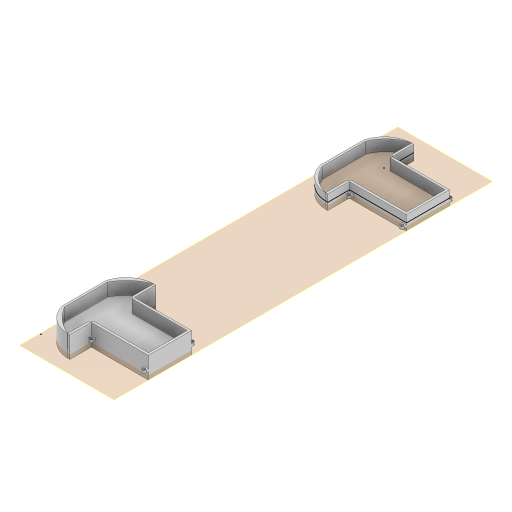
# Autodesk Inventor part: Part1
Saved by Autodesk Inventor 2024.3 (Build 283343000, 343)
## iProperties
Created: 2025-09-23
Part Number: Part1
Material: Generic
Document SubType Name: Modeling
Designer: danie
Density: 1 g/cm^3
Appearance: Default
Author: danie
Autodesk Inventor part; units mm, degrees
ref_plane "YZ Plane" through (0, 0, 0) normal (1, 0, 0) x (0, 1, 0)
ref_plane "XZ Plane" through (0, 0, 0) normal (0, 1, 0) x (-1, 0, 0)
ref_plane "XY Plane" through (0, 0, 0) normal (0, 0, 1) x (1, 0, 0)
sketch "Sketch1" plane through (0, 0, 0) normal (0, 1, 0) x (-1, 0, 0)
  line L0 (-60.8639, 0) -> (-200, 0)
  line L1 (-200, 0) -> (-200, -200)
  line L2 (-200, -200) -> (0, -200)
  line L3 (0, -200) -> (0, 0)
  line L4 (0, -200) -> (-200, -200)
  line L5 (-200, -200) -> (-200, -400)
  line L6 (-200, -400) -> (0, -400)
  line L7 (0, -400) -> (0, -200)
  line L8 (-60.8639, 0) -> (-67, 0)
  line L9 (0, -200) -> (0, -100)
  line L10 (0, -50) -> (0, -100)
  line L11 (0, -100) -> (0, -50)
  line L12 (0, -50) -> (0, -150)
  line L13 (0, -150) -> (-67, -150)
  line L14 (0, -50) -> (-67, -50)
  line L15 (-14.5617, -10.867) -> (0, 0)
  line L16 (-67, -150) -> (0, -200)
  arc A0 (0, -50) -> (-67, 0) centre (-63.932, -65.7788) ccw
  line L17 (0, -200) -> (15.754, -200)
  line L18 (15.754, -200) -> (0, -200)
  line L19 (0, -200) -> (0, -184.246)
  line L20 (0, -184.246) -> (-21.1104, -184.246)
  line L21 (-21.1104, -184.246) -> (-21.1104, -200)
  arc A1 (-67, -200) -> (0, -150) centre (-63.9339, -134.2186) ccw
  line L22 (-67, -50) -> (-200, -50)
  line L23 (-67, -150) -> (-200, -150)
  line L24 (-67, 0) -> (-67, -50)
  line L25 (-67, -150) -> (-67, -200)
  line L26 (-200, -800) -> (-200, -600)
  line L27 (0, -750) -> (0, -700)
  line L28 (0, -750) -> (0, -650)
  line L29 (0, -650) -> (-67, -650)
  line L30 (0, -750) -> (-67, -750)
  line L31 (-67, -650) -> (0, -600)
  arc A2 (-67, -800) -> (0, -750) centre (-63.932, -734.2212) ccw
  arc A3 (0, -650) -> (-67, -600) centre (-63.9339, -665.7814) ccw
  line L32 (-67, -750) -> (-200, -750)
  line L33 (-67, -650) -> (-200, -650)
  line L34 (-67, -800) -> (-67, -750)
  line L35 (-67, -650) -> (-67, -600)
  point P0 (-60.8677, -200)
  dimension "d0" = 200
  dimension "d1" = 200
  dimension "d2" = 200
  dimension "d3" = 200
  dimension "d4" = 67
  dimension "d5" = 100
  dimension "d6" = 50
  dimension "d7" = 100
  dimension "d8" = 15.754
  dimension "d9" = 15.754
  constraints: 72 end point, 14 symmetric about line, 13 perpendicular, 10 point on circle, 9 point on line, 4 centre point, 4 parallel, 2 collinear, 2 horizontal, 2 midpoint, 2 other
  measures "d0" distance of L2.end L1.end
  measures "d1" distance of L1.end L0.end
  measures "d2" distance of L6.end L5.end
  measures "d3" distance of L5.end L4.end
  measures "d4" distance of L3.end L8.end
  measures "d5" distance of L3.end L9.end
  measures "d6" distance of L10.start L9.end
  measures "d7" distance of L10.start L12.end
  measures "d8" distance of L2.end L17.end
  measures "d9" distance of L2.end L19.end
extrude "Extrusion1" add sketch "Sketch1" along normal blind 50 contours A0 L14 L24 L0 | L3 L13 L23 L1 L22 L14 | A1 L16 L13 | L16 A1 L2 L25 | L26 L33 L29 L28 L27 L30 L32 | L30 A2 L34 | L31 A3 L29 | L35 A3 L31
sketch "Sketch2" plane through (0, 50, 0) normal (0, 1, 0) x (1, 0, 0)
  line L0 (67, 50) -> (200, 50) projected
  line L1 (200, 50) -> (200, 150)
  line L2 (200, 150) -> (67, 150)
  line L3 (67, 150) -> (67, 199.2984)
  line L4 (67, 199.2984) -> (67, 200.0458)
  line L5 (0, 150) -> (0, 50) projected
  line L6 (0, 50) -> (0, 150)
  line L7 (67, 50) -> (200, 50)
  arc A0 (0, 50) -> (63.932, 0) centre (63.792, 65.694) ccw
  arc A1 (60.8677, 200) -> (0, 150) centre (63.9339, 134.2186) ccw projected
  arc A2 (67, 200.0458) -> (0, 150) centre (64.0367, 134.1412) ccw
  line L8 (107.1865, 50) -> (107.1865, 55)
  line L9 (107.1865, 55) -> (67, 55)
  line L10 (200, 55) -> (195, 55)
  line L11 (195, 150) -> (195, 145)
  line L12 (195, 145) -> (67, 145)
  line L13 (67, 145) -> (67, 55)
  line L14 (67, 55) -> (195, 55)
  line L15 (195, 55) -> (195, 145)
  line L16 (0, 102.5601) -> (5, 102.5601)
  line L17 (5, 102.5601) -> (5, 150)
  line L18 (67, 150) -> (67, 200) projected
  line L19 (67, 150) -> (62, 150)
  line L20 (62, 150) -> (5, 150)
  line L21 (62, 150) -> (62, 145)
  line L22 (62, 145) -> (72.629, 145)
  line L23 (67, 50) -> (62, 50)
  line L24 (62, 50) -> (62, 55)
  line L25 (62, 50) -> (5, 50)
  line L26 (5, 50) -> (5, 104.6986)
  line L27 (67, 55) -> (62, 55)
  line L28 (62, 50) -> (67, 55)
  line L29 (67, 145) -> (62, 150)
  line L30 (67, 200) -> (62.0007, 200.081)
  line L31 (62.0007, 200.081) -> (62, 150)
  arc A3 (62.0007, 200.081) -> (5, 150) centre (102.4081, 96.6117) ccw
  line L32 (62.0007, 50.0007) -> (62.0007, 0.0243)
  arc A4 (5, 50) -> (62.0007, 0.0243) centre (106.1149, 107.8339) ccw
  point P0 (0, 0)
  point P1 (62.0007, 50)
  dimension "d12" = 5
  dimension "d13" = 5
  dimension "d14" = 5
  dimension "d15" = 5
  dimension "d16" = 5
  dimension "d17" = 5
  dimension "d18" = 5
  constraints: 60 end point, 12 perpendicular, 10 point on circle, 9 point on line, 4 centre point, 4 horizontal, 2 collinear, 2 parallel, 2 vertical
  measures "d12" distance of L8.start L8.end
  measures "d13" distance of L10.start L10.end
  measures "d14" distance of L11.start L11.end
  measures "d15" distance of L16.start L16.end
  measures "d16" distance of L2.end L19.end
  measures "d17" distance of L0.start L23.end
  measures "d18" distance of L18.end L30.end
extrude "Extrusion2" cut sketch "Sketch2" against normal blind 30 contours L25 L26 L17 L20 L21 L22 L13 L27 L24 | L32 A4 L25 | L24 L27 L28 | L9 L13 L12 L15 L14 | L22 L21 L29 | L20 A3 L31
ref_plane "Work Plane1" through (0, 10, 0) normal (0, 1, 0) x (1, 0, 0)
sketch "Sketch3" plane through (0, 20, 0) normal (0, 1, 0) x (1, 0, 0)
  line L0 (67, 150) -> (200, 150) projected
  line L1 (200, 150) -> (200, 50) projected
  line L2 (200, 50) -> (67, 50) projected
  line L3 (67, 50) -> (67, 0) projected
  line L4 (67, 0) -> (60.8639, 0) projected
  arc A0 (0, 50) -> (60.8639, 0) centre (63.932, 65.7788) ccw projected
  line L5 (0, 50) -> (0, 150) projected
  arc A1 (60.8677, 200) -> (0, 150) centre (63.9339, 134.2186) ccw projected
  line L6 (60.8677, 200) -> (61.7939, 200) projected
  arc A2 (61.7939, 200) -> (5, 150) centre (102.4081, 96.6117) ccw projected
  line L7 (5, 150) -> (5, 50) projected
  arc A3 (5, 50) -> (62.0007, 0.0243) centre (106.1149, 107.8339) ccw projected
  line L8 (62.0007, 0.0243) -> (62.0007, 50) projected
  line L9 (62.0007, 50) -> (62, 50) projected
  line L10 (62, 50) -> (67, 55) projected
  line L11 (67, 55) -> (195, 55) projected
  line L12 (195, 55) -> (195, 145) projected
  line L13 (195, 145) -> (67, 145) projected
  line L14 (67, 145) -> (62, 150) projected
  line L15 (62, 150) -> (62.0007, 200) projected
  line L16 (61.7939, 200) -> (62.0007, 200) projected
  line L17 (67, 200) -> (67, 150) projected
  line L18 (62.0007, 200) -> (67, 200) projected
  arc A4 (0, 650) -> (67, 600) centre (63.9339, 665.7814) ccw projected
  line L19 (0, 650) -> (0, 750) projected
  arc A5 (67, 800) -> (0, 750) centre (63.932, 734.2212) ccw projected
  line L20 (67, 800) -> (67, 750) projected
  line L21 (67, 750) -> (200, 750) projected
  line L22 (200, 750) -> (200, 650) projected
  line L23 (200, 650) -> (67, 650) projected
  line L24 (67, 650) -> (67, 600) projected
  line L25 (67, 150) -> (200, 150) projected
  line L26 (200, 150) -> (200, 50) projected
  line L27 (200, 50) -> (67, 50) projected
  line L28 (67, 50) -> (67, 0) projected
  line L29 (67, 0) -> (60.8639, 0) projected
  arc A6 (0, 50) -> (60.8639, 0) centre (63.932, 65.7788) ccw projected
  line L30 (0, 50) -> (0, 150) projected
  arc A7 (60.8677, 200) -> (0, 150) centre (63.9339, 134.2186) ccw projected
  line L31 (60.8677, 200) -> (61.7939, 200) projected
  arc A8 (61.7939, 200) -> (5, 150) centre (102.4081, 96.6117) ccw projected
  line L32 (5, 150) -> (5, 50) projected
  arc A9 (5, 50) -> (62.0007, 0.0243) centre (106.1149, 107.8339) ccw projected
  line L33 (62.0007, 0.0243) -> (62.0007, 50) projected
  line L34 (62.0007, 50) -> (62, 50) projected
  line L35 (62, 50) -> (67, 55) projected
  line L36 (67, 55) -> (195, 55) projected
  line L37 (195, 55) -> (195, 145) projected
  line L38 (195, 145) -> (67, 145) projected
  line L39 (67, 145) -> (62, 150) projected
  line L40 (62, 150) -> (62.0007, 200) projected
  line L41 (61.7939, 200) -> (62.0007, 200) projected
  line L42 (67, 200) -> (67, 150) projected
  line L43 (62.0007, 200) -> (67, 200) projected
  arc A10 (0, 650) -> (67, 600) centre (63.9339, 665.7814) ccw projected
  line L44 (0, 650) -> (0, 750) projected
  arc A11 (67, 800) -> (0, 750) centre (63.932, 734.2212) ccw projected
  line L45 (67, 800) -> (67, 750) projected
  line L46 (67, 750) -> (200, 750) projected
  line L47 (200, 750) -> (200, 650) projected
  line L48 (200, 650) -> (67, 650) projected
  line L49 (67, 650) -> (67, 600) projected
  line L50 (67, 50) -> (200, 50) projected
  line L51 (67, 50) -> (77, 50)
  line L52 (77, 50) -> (77, 40)
  line L53 (77, 40) -> (67, 40)
  line L54 (67, 40) -> (67, 50)
  line L55 (200, 50) -> (190, 50)
  line L56 (190, 50) -> (190, 40)
  line L57 (190, 40) -> (200, 40)
  line L58 (200, 40) -> (200, 50)
  line L59 (200, 50) -> (200, 150) projected
  line L60 (200, 150) -> (190, 150)
  line L61 (190, 150) -> (190, 160)
  line L62 (190, 160) -> (200, 160)
  line L63 (200, 160) -> (200, 150)
  line L64 (67, 150) -> (77, 150)
  line L65 (77, 150) -> (77, 160)
  line L66 (77, 160) -> (67, 160)
  line L67 (67, 160) -> (67, 150)
  circle A12 centre (72, 45) radius 5
  circle A13 centre (195, 45) radius 5
  circle A14 centre (195, 155) radius 5
  circle A15 centre (72, 155) radius 5
  point P0 (0, 0)
  point P1 (67, 45)
  point P2 (77, 45)
  point P3 (190, 45)
  point P4 (200, 45)
  point P5 (190, 155)
  point P6 (200, 155)
  point P7 (77, 155)
  point P8 (67, 155)
  dimension "d21" = 10
  dimension "d22" = 10
  dimension "d23" = 10
  dimension "d24" = 10
  dimension "d25" = 10
  dimension "d26" = 10
  dimension "d27" = 10
  constraints: 32 end point, 8 parallel, 4 centre point, 4 horizontal, 4 perpendicular
  measures "d21" distance of L52.end L53.end
  measures "d22" distance of L51.end L52.end
  measures "d23" distance of L57.end L56.end
  measures "d24" distance of L56.end L55.end
  measures "d25" distance of L61.end L62.end
  measures "d26" distance of L60.end L61.end
  measures "d27" distance of L66.end L65.end
extrude "Extrusion3" add sketch "Sketch3" along normal mid plane 5.75 contours L0 A15 L65 | L61 A14 L0 | L0 L17 A15 | A15 | A14 L63 L0 | A14 | L58 A13 L2 | A13 L56 L2 | A13 | L52 A12 L2 | A12 L3 L2 | A12
sketch "Sketch4" plane through (0, 22.875, 0) normal (0, 1, 0) x (1, 0, 0)
  circle A0 centre (72, 44.2688) radius 3.375
  arc A1 (190, 45) -> (200, 45) centre (195, 45) ccw projected
  line L0 (195, 40) -> (195, 44.2688)
  circle A2 centre (195, 44.2688) radius 3.375
  arc A3 (200, 155) -> (190, 155) centre (195, 155) ccw projected
  line L1 (195, 160) -> (195, 155.731)
  circle A4 centre (195, 155.731) radius 2.875
  circle A5 centre (195, 155.731) radius 3.375
  arc A6 (77, 155) -> (67, 155) centre (72, 155) ccw projected
  line L2 (72, 160) -> (72, 155.731)
  circle A7 centre (72, 155.731) radius 3.375
  point P0 (0, 0)
  dimension "d30" = 6.75
  dimension "d31" = 4.269
  dimension "d32" = 5.75
  dimension "d33" = 6.75
  constraints: 6 end point, 5 centre point, 4 coincident, 3 point on circle, 3 vertical
  measures "d30" diameter of A0
  measures "d31" distance of L1.start L1.end
  measures "d32" diameter of A4
  measures "d33" diameter of A5
extrude "Extrusion4" cut sketch "Sketch4" against normal blind 5.75 contours A0 | A2 | A4 | A5 | A7
thread "Thread1" size "M7x1" class "6H" standard "ANSI Metric M Profile" full length
thread "Thread2" size "M7x1" class "6H" standard "ANSI Metric M Profile" full length
thread "Thread3" size "M7x1" class "6H" standard "ANSI Metric M Profile" full length
thread "Thread4" size "M7x1" class "6H" standard "ANSI Metric M Profile" full length
sketch "Sketch5" plane through (0, 17.125, 0) normal (0, -1, 0) x (1, 0, 0)
  line L0 (200, -750) -> (67, -750)
  line L1 (67, -750) -> (200, -750)
  line L2 (200, -750) -> (200, -650.0001)
  line L3 (200, -650.0001) -> (67, -650.0001)
  line L4 (67, -600) -> (67, -650)
  line L5 (0, -750) -> (0, -650)
  arc A0 (67, -600) -> (0, -650) centre (63.2865, -664.914) ccw
  arc A1 (0, -750) -> (67, -800) centre (63.932, -734.2212) ccw
  arc A2 (0, -750) -> (67, -800) centre (63.932, -734.2212) ccw
  line L6 (0, -650) -> (0, -750)
  line L7 (67, -750) -> (67, -800)
  line L8 (67, -600) -> (67, -650)
  point P0 (0, 0)
  constraints: 18 end point, 6 point on circle, 3 centre point
sketch "Sketch6" plane through (0, 50, 0) normal (0, 1, 0) x (1, 0, 0)
  arc A0 (0, 650) -> (67, 600) centre (63.9339, 665.7814) ccw projected
  line L0 (0, 750) -> (0, 650) projected
  line L1 (0, 650) -> (0, 750)
  line L2 (67, 650) -> (200, 650) projected
  line L3 (67, 650) -> (200, 650)
  line L4 (200, 650) -> (200, 750)
  line L5 (200, 750) -> (67, 750)
  line L6 (67, 750) -> (67, 800)
  line L7 (67, 600) -> (67, 650) projected
  line L8 (67, 650) -> (67, 600)
  arc A1 (0, 650) -> (67, 600) centre (63.9339, 665.7814) ccw
  arc A2 (67, 800) -> (0, 750) centre (63.932, 734.2212) ccw projected
  arc A3 (67, 800) -> (0, 750) centre (63.932, 734.2212) ccw
  point P0 (0, 0)
  dimension "d44" = 50
  constraints: 12 end point, 4 point on circle, 3 perpendicular, 2 centre point, 1 collinear, 1 concentric, 1 horizontal, 1 vertical
  measures "d44" distance of L5.end L6.end
extrude "Extrusion5" cut sketch "Sketch6" against normal blind 16.5
sketch "Sketch7" plane through (0, 33.5, 0) normal (0, 1, 0) x (1, 0, 0)
  line L0 (200, 750) -> (67, 750) projected
  line L1 (200, 750) -> (200, 745)
  line L2 (0, 750) -> (0, 650) projected
  line L3 (200, 745) -> (195, 745)
  line L4 (67, 650) -> (200, 650) projected
  line L5 (195, 650) -> (195, 655)
  line L6 (195, 655) -> (67, 655)
  line L7 (195, 655) -> (195, 745)
  line L8 (200, 650) -> (200, 750) projected
  line L9 (195, 745) -> (67, 745)
  line L10 (67, 745) -> (67, 655)
  line L11 (67, 800.7968) -> (62, 800.7968)
  line L12 (62, 800.7968) -> (62, 600)
  line L13 (67, 650) -> (67, 655)
  line L14 (67, 655) -> (62, 650)
  line L15 (67, 750) -> (62, 755)
  line L16 (0, 750) -> (5, 750)
  arc A0 (67, 800) -> (0, 750) centre (63.932, 734.2212) ccw projected
  line L17 (62, 800.0432) -> (65.8623, 800.1565)
  line L18 (65.8623, 800.1565) -> (67, 800)
  line L19 (67, 800) -> (62, 800.0432)
  line L20 (67, 800) -> (67, 750)
  line L21 (0, 750) -> (0, 650)
  line L22 (0, 650) -> (5, 650)
  line L23 (5, 650) -> (5, 750)
  arc A1 (62, 800.0432) -> (5, 750) centre (81.2834, 720.5955) ccw
  line L24 (62, 650) -> (62, 600)
  arc A2 (0, 650) -> (67, 600) centre (63.9339, 665.7814) ccw projected
  line L25 (62, 600) -> (67, 600)
  line L26 (67, 600) -> (67, 600)
  line L27 (67, 650) -> (67, 600)
  arc A3 (5, 650) -> (62, 600) centre (82.4475, 680.8001) ccw
  line L28 (67, 750) -> (67, 650)
  point P0 (0, 0)
  dimension "d47" = 5
  dimension "d48" = 5
  dimension "d49" = 5
  dimension "d50" = 5
  dimension "d51" = 5
  constraints: 50 end point, 8 perpendicular, 5 point on circle, 5 point on line, 4 horizontal, 4 parallel, 2 centre point, 2 vertical, 1 tangent
  measures "d47" distance of L0.start L1.end
  measures "d48" distance of L1.end L3.end
  measures "d49" distance of L5.start L5.end
  measures "d50" distance of L11.start L11.end
  measures "d51" distance of L2.start L16.end
extrude "Extrusion6" cut sketch "Sketch7" against normal blind 25.75 contours L28 L10 L14 L12 L15 | L12 A3 L23 A1 | L9 L7 L6 L10
sketch "Sketch8" plane through (0, 10, 0) normal (0, 1, 0) x (1, 0, 0)
  line L0 (61.7939, 200) -> (62.0007, 200) projected
  arc A0 (61.7939, 200) -> (5, 150) centre (102.4081, 96.6117) ccw projected
  line L1 (5, 50) -> (5, 150) projected
  arc A1 (5, 50) -> (62.0007, 0.0243) centre (106.1149, 107.8339) ccw projected
  line L2 (62.0007, 50) -> (62.0007, 0.0243) projected
  line L3 (62, 50) -> (62.0007, 50) projected
  line L4 (67, 55) -> (62, 50) projected
  line L5 (195, 55) -> (67, 55) projected
  line L6 (195, 145) -> (195, 55) projected
  line L7 (67, 145) -> (195, 145) projected
  line L8 (62, 150) -> (67, 145) projected
  line L9 (62.0007, 200) -> (62, 150) projected
  line L10 (67, 650) -> (67, 600) projected
  arc A2 (0, 650) -> (67, 600) centre (63.9339, 665.7814) ccw projected
  line L11 (0, 650) -> (0, 750) projected
  arc A3 (67, 800) -> (62, 800.0432) centre (63.932, 734.2212) ccw projected
  arc A4 (62, 800.0432) -> (5, 750) centre (81.2834, 720.5955) ccw projected
  line L12 (5, 750) -> (5, 650) projected
  arc A5 (5, 650) -> (62, 600) centre (82.4475, 680.8001) ccw projected
  line L13 (62, 600) -> (62, 650) projected
  line L14 (62, 650) -> (67, 655) projected
  line L15 (67, 655) -> (195, 655) projected
  line L16 (195, 655) -> (195, 745) projected
  line L17 (195, 745) -> (67, 745) projected
  line L18 (67, 745) -> (67, 750) projected
  line L19 (67, 800) -> (67, 750) projected
  arc A6 (62, 800.0432) -> (0, 750) centre (63.932, 734.2212) ccw projected
  line L20 (62, 755) -> (62, 800.0432) projected
  line L21 (67, 750) -> (62, 755) projected
  line L22 (67, 750) -> (200, 750) projected
  line L23 (200, 750) -> (200, 650) projected
  line L24 (200, 650) -> (67, 650) projected
  line L25 (67, 150) -> (200, 150) projected
  line L26 (200, 150) -> (200, 50) projected
  line L27 (200, 50) -> (67, 50) projected
  line L28 (67, 50) -> (67, 0) projected
  line L29 (67, 0) -> (60.8639, 0) projected
  arc A7 (0, 50) -> (60.8639, 0) centre (63.932, 65.7788) ccw projected
  line L30 (0, 50) -> (0, 150) projected
  arc A8 (60.8677, 200) -> (0, 150) centre (63.9339, 134.2186) ccw projected
  line L31 (60.8677, 200) -> (67, 200) projected
  line L32 (67, 200) -> (67, 150) projected
  line L33 (67, 650) -> (67, 600) projected
  arc A9 (0, 650) -> (67, 600) centre (63.9339, 665.7814) ccw projected
  line L34 (0, 650) -> (0, 750) projected
  arc A10 (67, 800) -> (62, 800.0432) centre (63.932, 734.2212) ccw projected
  arc A11 (62, 800.0432) -> (5, 750) centre (81.2834, 720.5955) ccw projected
  line L35 (5, 750) -> (5, 650) projected
  arc A12 (5, 650) -> (62, 600) centre (82.4475, 680.8001) ccw projected
  line L36 (62, 600) -> (62, 650) projected
  line L37 (62, 650) -> (67, 655) projected
  line L38 (67, 655) -> (195, 655) projected
  line L39 (195, 655) -> (195, 745) projected
  line L40 (195, 745) -> (67, 745) projected
  line L41 (67, 745) -> (67, 750) projected
  line L42 (67, 800) -> (67, 750) projected
  arc A13 (62, 800.0432) -> (0, 750) centre (63.932, 734.2212) ccw projected
  line L43 (62, 755) -> (62, 800.0432) projected
  line L44 (67, 750) -> (62, 755) projected
  line L45 (67, 750) -> (200, 750) projected
  line L46 (200, 750) -> (200, 650) projected
  line L47 (200, 650) -> (67, 650) projected
  line L48 (67, 150) -> (200, 150) projected
  line L49 (200, 150) -> (200, 50) projected
  line L50 (200, 50) -> (67, 50) projected
  line L51 (67, 50) -> (67, 0) projected
  line L52 (67, 0) -> (60.8639, 0) projected
  arc A14 (0, 50) -> (60.8639, 0) centre (63.932, 65.7788) ccw projected
  line L53 (0, 50) -> (0, 150) projected
  arc A15 (60.8677, 200) -> (0, 150) centre (63.9339, 134.2186) ccw projected
  line L54 (60.8677, 200) -> (67, 200) projected
  line L55 (67, 200) -> (67, 150) projected
  line L56 (67, 650) -> (77, 650)
  line L57 (77, 650) -> (77, 640)
  line L58 (77, 640) -> (67, 640)
  line L59 (67, 640) -> (67, 650)
  line L60 (200, 650) -> (190, 650)
  line L61 (190, 650) -> (190, 640)
  line L62 (190, 640) -> (200, 640)
  line L63 (200, 640) -> (200, 650)
  line L64 (67, 750) -> (77, 750)
  line L65 (77, 750) -> (77, 760)
  line L66 (77, 760) -> (67, 760)
  line L67 (67, 760) -> (67, 750)
  line L68 (200, 750) -> (190, 750)
  line L69 (190, 750) -> (190, 760)
  line L70 (190, 760) -> (200, 760)
  line L71 (200, 760) -> (200, 750)
  circle A16 centre (72, 755) radius 5
  circle A17 centre (195, 755) radius 5
  circle A18 centre (72, 645) radius 5
  circle A19 centre (195, 645) radius 5
  point P0 (0, 0)
  point P1 (77, 755)
  point P2 (67, 755)
  point P3 (200, 755)
  point P4 (190, 755)
  point P5 (190, 645)
  point P6 (200, 645)
  point P7 (67, 645)
  point P8 (77, 645)
  dimension "d54" = 10
  dimension "d55" = 10
  dimension "d56" = 10
  dimension "d57" = 10
  dimension "d58" = 10
  dimension "d59" = 10
  constraints: 32 end point, 8 parallel, 4 centre point, 4 horizontal, 4 perpendicular, 2 point on line
  measures "d54" distance of L57.end L58.end
  measures "d55" distance of L56.end L57.end
  measures "d56" distance of L62.end L61.end
  measures "d57" distance of L61.end L60.end
  measures "d58" distance of L66.end L65.end
  measures "d59" distance of L65.end L64.end
extrude "Extrusion7" add sketch "Sketch8" along normal mid plane 5.75 contours L10 L24 A18 | A18 | L24 L57 A18 | L24 A19 L61 | L24 L63 A19 | A19 | L19 A16 L22 | A16 | A16 L65 L22 | L22 A17 L71 | L22 L69 A17 | A17
sketch "Sketch9" plane through (0, 12.875, 0) normal (0, 1, 0) x (1, 0, 0)
  arc A0 (67, 645) -> (77, 645) centre (72, 645) ccw projected
  line L0 (72, 640) -> (72, 644.269)
  circle A1 centre (72, 644.269) radius 3.375
  arc A2 (190, 645) -> (200, 645) centre (195, 645) ccw projected
  line L1 (195, 640) -> (195, 644.269)
  circle A3 centre (195, 644.269) radius 3.375
  arc A4 (200, 755) -> (190, 755) centre (195, 755) ccw projected
  line L2 (195, 760) -> (195, 755.731)
  circle A5 centre (195, 755.731) radius 3.375
  line L3 (72, 760) -> (72, 755.731)
  circle A6 centre (72, 755.731) radius 3.375
  point P0 (0, 0)
  dimension "d62" = 4.269
  dimension "d63" = 6.75
  dimension "d64" = 4.269
  dimension "d65" = 6.75
  constraints: 8 end point, 4 centre point, 4 coincident, 4 vertical, 3 point on circle
  measures "d62" distance of L0.start L0.end
  measures "d63" diameter of A1
  measures "d64" distance of L2.start L2.end
  measures "d65" diameter of A5
extrude "Extrusion8" cut sketch "Sketch9" against normal blind 5.75
thread "Thread5" size "M7x1" class "6H" standard "ANSI Metric M Profile" full length
thread "Thread6" size "M7x1" class "6H" standard "ANSI Metric M Profile" full length
thread "Thread7" size "M7x1" class "6H" standard "ANSI Metric M Profile" full length
thread "Thread8" size "M7x1" class "6H" standard "ANSI Metric M Profile" full length
sketch "Sketch10" plane through (200, 0, -150) normal (0, 0, -1) x (-1, 0, 0)
  point P0 (200, 0)
body "Solid1"
